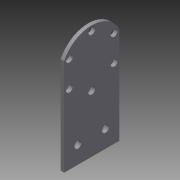
# Autodesk Inventor part: Hub Mount Plate
Saved by Autodesk Inventor 2014 SP1 (Build 180222100, 222)
## iProperties
Created: 2014-01-16
Part Number: Hub Mount Plate
Material: Generic
Document SubType Name: Modeling
Designer: JU BRIAN
Density: 1 g/cm^3
Appearance: Default
Author: JU BRIAN
Autodesk Inventor part; units mm, degrees
ref_plane "YZ Plane" through (0, 0, 0) normal (1, 0, 0) x (0, 1, 0)
ref_plane "XZ Plane" through (0, 0, 0) normal (0, 1, 0) x (-1, 0, 0)
ref_plane "XY Plane" through (0, 0, 0) normal (0, 0, 1) x (1, 0, 0)
sketch "Sketch1" plane through (0, 0, 0) normal (1, 0, 0) x (0, 1, 0)
  line L0 (45.5354, 147.0574) -> (-5.2646, 147.0574)
  line L1 (-5.2646, 147.0574) -> (-5.2646, 58.1574)
  arc A0 (-5.2646, 58.1574) -> (45.5354, 58.1574) centre (20.1354, 70.5399) ccw
  line L2 (45.5354, 147.0574) -> (45.5354, 58.1574)
  point P0 (20.1354, 42.2824)
  dimension "d0" = 50.8
  dimension "d1" = 88.9
  dimension "d2" = 15.875
  constraints: 6 end point, 3 point on circle, 1 centre point, 1 parallel, 1 perpendicular
  measures "d0" distance of L0.start L0.end
  measures "d1" distance of L0.end L1.end
  measures "d2" vertical distance of L2.end point (20.135, 42.282)
extrude "Extrusion1" add sketch "Sketch1" along normal blind 3.175
sketch "Sketch2" plane through (3.175, 0, 0) normal (1, 0, 0) x (0, 0, -1)
  line L0 (-147.0574, 45.5354) -> (-147.0574, -5.2646) projected
  line L1 (-82.4462, 40.7576) -> (-58.6337, -0.4869)
  point P0 (-82.4462, 40.7576)
  point P1 (-94.3524, 20.1354)
  point P2 (-58.6337, 40.7576)
  point P3 (-46.7274, 20.1354)
  point P4 (-58.6337, -0.4869)
  point P5 (-82.4462, -0.4869)
  dimension "d5" = 47.625
  dimension "d6" = 30
  constraints: 2 end point
  measures "d5" distance of L1.start L1.end
  measures "d6" angle of L0 L1
hole "Hole1" at (3.175, 40.7576, 82.4462) at (3.175, 20.1354, 94.3524) at (3.175, 40.7576, 58.6337) at (3.175, 20.1354, 46.7274) at (3.175, -0.4869, 58.6337) at (3.175, -0.4869, 82.4462) direction (-1, 0, 0) diameter 6.35 end through all
sketch "Sketch3" plane through (3.175, 0, 0) normal (1, 0, 0) x (0, 0, -1)
  line L0 (-147.0574, 45.5354) -> (-147.0574, -5.2646) projected
  line L1 (-58.1574, 45.5354) -> (-147.0574, 45.5354) projected
  point P0 (-131.1824, 32.8354)
  point P1 (-131.1824, 7.4354)
  dimension "d18" = 25.4
  dimension "d19" = 12.7
  dimension "d20" = 15.875
  constraints: 1 vertical alignment
  measures "d18" distance of point (-131.182, 32.835) point (-131.182, 7.435)
  measures "d19" distance from line of L1 point (-131.182, 32.835)
  measures "d20" distance from line of L0 point (-131.182, 7.435)
hole "Hole2" at (3.175, 32.8354, 131.1824) at (3.175, 7.4354, 131.1824) direction (-1, 0, 0) diameter 6.35 end through all
body "Solid1"
